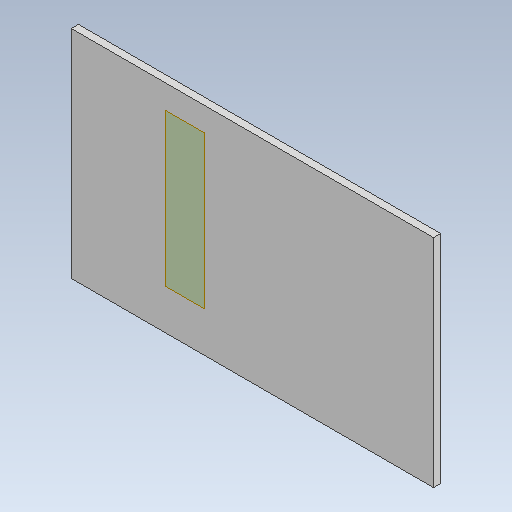
# Autodesk Inventor part: placa
Saved by Autodesk Inventor 2021 (Build 250183000, 183)
## iProperties
Created: 2021-06-18
Part Number: placa
Material: Generic
Document SubType Name: Modeling
Designer: Andrés Holguín
Density: 1 g/cm^3
Appearance: Default
Author: Andrés Holguín
Autodesk Inventor part; units mm, degrees
ref_plane "YZ Plane" through (0, 0, 0) normal (1, 0, 0) x (0, 1, 0)
ref_plane "XZ Plane" through (0, 0, 0) normal (0, 1, 0) x (-1, 0, 0)
ref_plane "XY Plane" through (0, 0, 0) normal (0, 0, 1) x (1, 0, 0)
ref_plane "Work Plane1" through (163.8833, 172.5103, 148.8088) normal (0, 0, -1) x (-1, 0, 0)
sketch "Sketch1" plane through (163.8833, 172.5103, 148.8088) normal (0, 0, -1) x (-1, 0, 0)
  line L0 (-373.5501, 499.0968) -> (133.8917, 499.0968)
  line L1 (133.8917, 499.0968) -> (133.8917, 195.8448)
  line L2 (133.8917, 195.8448) -> (-373.5501, 195.8448)
  line L3 (-373.5501, 195.8448) -> (-373.5501, 499.0968)
  point P0 (163.8833, -172.5103)
  constraints: 8 end point, 2 parallel, 1 horizontal, 1 perpendicular
extrude "Extrusion1" add sketch "Sketch1" along normal blind 10
body "Solid1"
